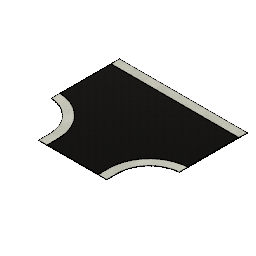
_T Section - Ruby.ac228448-3f17-452c-b31e-1589550a6ac2 (Autodesk Fusion 360 design; units mm, degrees)
Autodesk Fusion 360 part; units mm, degrees
sketch "Sketch1" plane through (0, 0, 0) normal (0, 0, 1) x (1, 0, 0)
  line L0 (0, 0) -> (1524, 0)
  line L1 (1524, 0) -> (1524, -609.6)
  line L2 (1524, -609.6) -> (0, -609.6)
  line L3 (0, -609.6) -> (0, 0)
  line L4 (1066.8, -304.8) -> (457.2, -304.8)
  line L5 (457.2, -304.8) -> (457.2, -914.4)
  line L6 (457.2, -914.4) -> (1066.8, -914.4)
  line L7 (1066.8, -914.4) -> (1066.8, -304.8)
  line L8 (1066.8, -304.8) -> (457.2, -914.4) construction
  line L9 (457.2, -304.8) -> (1066.8, -914.4) construction
  line L10 (457.2, -914.4) -> (1066.8, -914.4)
  line L11 (1066.8, -914.4) -> (1066.8, -1219.2)
  line L12 (1066.8, -1219.2) -> (457.2, -1219.2)
  line L13 (457.2, -1219.2) -> (457.2, -914.4)
  point P0 (762, -609.6)
  dimension "d1" = 1524
  dimension "d2" = 609.6
  dimension "d3" = 609.6
  dimension "d4" = 609.6
  dimension "d5" = 609.6
  dimension "d6" = 304.8
  constraint horizontal L0
  constraint vertical L1
  constraint horizontal L2
  constraint vertical L3
  constraint coincident L0.start L3.end
  constraint horizontal L4
  constraint perpendicular L4 L5
  constraint parallel L4 L6
  constraint parallel L5 L7
  constraint coincident L8 P0
  constraint coincident L9 P0
  constraint midpoint L2 P0
  constraint horizontal L10
  constraint vertical L11
  constraint horizontal L12
  constraint vertical L13
  measures "d1" distance of L0.start L0.end
  measures "d2" distance of L0.start L2.end
  measures "d3" distance of L5.end L6.end
  measures "d4" distance of L4.end L5.end
  measures "d5" distance of L5.end L6.end
  measures "d6" distance of L5.end L12.end
extrude "Extrude1" add sketch "Sketch1" along normal blind 6.35 makes body 1
fillet "Fillet1" radius 482.6 1 edges at (1066.8, -609.6, 3.175) on bodies 1
fillet "Fillet2" radius 482.6 1 edges at (457.2, -609.6, 3.175) on bodies 1
sketch "Sketch2" plane through (0, 0, 6.35) normal (0, 0, 1) x (-1, 0, 0)
  line L0 (-1524, 609.6) -> (-1524, 0)
  line L1 (-1524, 0) -> (0, 0)
  line L2 (0, 0) -> (0, 609.6)
  arc A0 (-457.2, 1091.5311) -> (0, 609.6) centre (25.4, 1091.5311) ccw
  line L3 (-457.2, 1091.5311) -> (-457.2, 1219.2)
  line L4 (-457.2, 1219.2) -> (-1066.8, 1219.2)
  line L5 (-1066.8, 1219.2) -> (-1066.8, 1091.5311)
  arc A1 (-1524, 609.6) -> (-1066.8, 1091.5311) centre (-1549.4, 1091.5311) ccw
  arc A2 (-355.6, 1091.5311) -> (101.6, 718.2289) centre (25.4, 1091.5311) ccw
  line L6 (101.6, -101.6) -> (101.6, 718.2289)
  line L7 (-1625.6, -101.6) -> (101.6, -101.6)
  line L8 (-1625.6, 718.2289) -> (-1625.6, -101.6)
  arc A3 (-1625.6, 718.2289) -> (-1168.4, 1091.5311) centre (-1549.4, 1091.5311) ccw
  line L9 (-1168.4, 1320.8) -> (-1168.4, 1091.5311)
  line L10 (-355.6, 1320.8) -> (-1168.4, 1320.8)
  line L11 (-355.6, 1091.5311) -> (-355.6, 1320.8)
  line L12 (101.6, 718.2289) -> (0, 718.2289)
  line L13 (0, 718.2289) -> (0, -101.6)
  line L14 (0, -101.6) -> (101.6, -101.6)
  line L15 (101.6, -101.6) -> (101.6, 718.2289)
  line L16 (-1625.6, 718.2289) -> (-1524, 718.2289)
  line L17 (-1524, 718.2289) -> (-1524, -101.6)
  line L18 (-1524, -101.6) -> (-1625.6, -101.6)
  line L19 (-1625.6, -101.6) -> (-1625.6, 718.2289)
  line L20 (-355.6, 1320.8) -> (-1168.4, 1320.8)
  line L21 (-1168.4, 1320.8) -> (-1168.4, 1219.2)
  line L22 (-1168.4, 1219.2) -> (-355.6, 1219.2)
  line L23 (-355.6, 1219.2) -> (-355.6, 1320.8)
  dimension "d13" = 101.6
  dimension "d14" = 101.6
  dimension "d15" = 101.6
  constraint horizontal L12
  constraint vertical L13
  constraint horizontal L14
  constraint vertical L15
  constraint coincident L7 L13.end
  constraint horizontal L16
  constraint vertical L17
  constraint horizontal L18
  constraint vertical L19
  constraint horizontal L20
  constraint vertical L21
  constraint horizontal L22
  constraint vertical L23
  measures "d14" distance of L8.start L16.end
  measures "d15" distance of L10.start L22.end
extrude "Extrude1'" add sketch "Sketch2" against normal blind 6.35 separate body contours L5 A1 A3 L9 L17 L22 | L1 L7 L13 L17 | A0 L3 A2 L11 L13 L22 makes body 2 at (389.4667, -1176.6437, 6.35) makes body 3 at (1016, 33.8667, 6.35) makes body 4 at (1134.5333, -1134.0874, 6.35) in component "T Intersection"
copy_body "CutPasteBodies1" bodies 1 removing the originals makes body 5 in component "T Intersection"
component "T Intersection" placed x (1, 0, 0) y (0, 1, 0) z (0, 0, 1) at (0, 0, 0)
